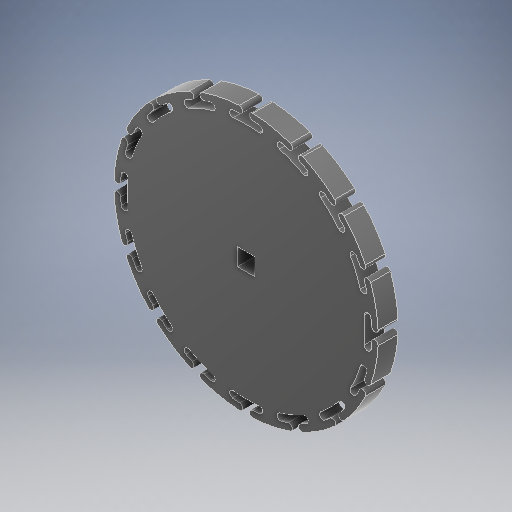
# Autodesk Inventor part: CustomRoller-01
Saved by Autodesk Inventor 2026.1 (Build 301233000, 233)
## iProperties
Created: 2025-10-16
Part Number: CustomRoller-01
Material: Plastic, Opaque Black
Document SubType Name: Modeling
Designer: Teddy
Density: 0.952 g/cm^3
Appearance: Smooth - Black
Diam: 2.000 in
HighStength: False
Author: Teddy
Autodesk Inventor part; units mm, degrees
ref_plane "YZ Plane" through (0, 0, 0) normal (1, 0, 0) x (0, 1, 0)
ref_plane "XZ Plane" through (0, 0, 0) normal (0, 1, 0) x (-1, 0, 0)
ref_plane "XY Plane" through (0, 0, 0) normal (0, 0, 1) x (1, 0, 0)
sketch "Sketch1" plane through (0, 0, 0) normal (0, 0, 1) x (1, 0, 0)
  circle A0 centre (0, 0) radius 25.4
  line L0 (-1.651, -1.651) -> (1.651, -1.651)
  line L1 (1.651, -1.651) -> (1.651, 1.651)
  line L2 (1.651, 1.651) -> (-1.651, 1.651)
  line L3 (-1.651, 1.651) -> (-1.651, -1.651)
  line L4 (-1.651, -1.651) -> (1.651, 1.651) construction
  line L5 (1.651, -1.651) -> (-1.651, 1.651) construction
  dimension "Diam_Sketch" = 50.8
  dimension "LowStrengthWidth" = 3.302
  constraints: 12 end point, 2 midpoint, 2 parallel, 2 perpendicular, 1 centre point, 1 coincident, 1 horizontal
  measures "Diam_Sketch" diameter of A0
  measures "LowStrengthWidth" distance of L1.end L2.end
extrude "Extrusion1" add sketch "Sketch1" along normal blind 3.81
sketch "Sketch2" plane through (0, 0, 3.81) normal (0, 0, 1) x (1, 0, 0)
  line L0 (-3.302, -3.302) -> (3.302, -3.302)
  line L1 (3.302, -3.302) -> (3.302, 3.302)
  line L2 (3.302, 3.302) -> (-3.302, 3.302)
  line L3 (-3.302, 3.302) -> (-3.302, -3.302)
  line L4 (-3.302, -3.302) -> (3.302, 3.302) construction
  line L5 (3.302, -3.302) -> (-3.302, 3.302) construction
  point P0 (0, 0)
  dimension "HighStrengthWidth" = 6.604
  constraints: 12 end point, 2 midpoint, 2 parallel, 2 perpendicular, 1 horizontal
  measures "HighStrengthWidth" distance of L1.end L2.end
extrude "HighStrenthCut" [suppressed]
sketch "Sketch3" plane through (0, 0, 3.81) normal (0, 0, 1) x (1, 0, 0)
  circle A0 centre (0, 0) radius 23.495 construction
  arc A1 (2.54, 23.3573) -> (-2.54, 23.3573) centre (0, 0) ccw construction
  arc A2 (2.6086, 23.9886) -> (-2.6086, 23.9886) centre (0, 0) ccw
  arc A3 (2.4714, 22.726) -> (-2.4714, 22.726) centre (0, 0) ccw
  arc A4 (2.4714, 22.726) -> (2.6086, 23.9886) centre (2.54, 23.3573) ccw
  arc A5 (-2.6086, 23.9886) -> (-2.4714, 22.726) centre (-2.54, 23.3573) ccw
  line L0 (-2.54, 23.3573) -> (0, 0) construction
  line L1 (0, 0) -> (2.54, 23.3573) construction
  line L2 (0, 0) -> (0, 23.495) construction
  arc A6 (-1.2374, 24.0982) -> (-1.3026, 25.3666) centre (-1.27, 24.7324) ccw
  arc A7 (1.3026, 25.3666) -> (1.2374, 24.0982) centre (1.27, 24.7324) ccw
  circle A8 centre (0, 0) radius 25.4 projected
  arc A9 (-1.336, 26.67) -> (-1.3026, 25.3666) centre (-1.336, 26.0179) ccw
  line L3 (-1.336, 26.67) -> (1.336, 26.67)
  arc A10 (1.3026, 25.3666) -> (1.336, 26.67) centre (1.336, 26.0179) ccw
  dimension "ToothDiam" = 46.99
  dimension "ToothLength" = 5.08
  dimension "ToothWidth" = 1.27
  dimension "OutsideCut" = 26.67
  constraints: 21 point on circle, 13 tangent, 9 centre point, 8 end point, 2 coincident, 1 equal radius, 1 horizontal, 1 symmetric about line, 1 vertical, 5 other
  measures "ToothLength" distance of L1.end L0.start
  measures "OutsideCut" distance from line of A8.centre L3
extrude "Extrusion3" cut sketch "Sketch3" against normal blind 3.81 contours A4 A3 A5 A2 | A2 A6 A8 A7 | A8 A9 L3 A10
pattern_circular "Circular Pattern1" count 16 over 360 about axis through (0, 0, 0) along (0, 0, 1) of "Extrusion3"
equation "\"Diam_Sketch\" = Diam"
equation "\"HighStrengthCutDepth\" = SprocketWidth"
equation "\"ToothDepth\" = SprocketWidth"
equation "\"Diam\" = 50.8"
equation "\"SprocketWidth\" = 3.81"
body "Solid1"
